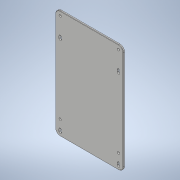
# Autodesk Inventor part: TBD_Box_Fix
Saved by Autodesk Inventor 2021 (Build 250183000, 183)
## iProperties
Created: 2020-10-24
Part Number: TBD_Box_Fix
Material: Generic
Document SubType Name: Modeling
Designer: lgnds
Density: 1 g/cm^3
Appearance: Default
Author: lgnds
Autodesk Inventor part; units mm, degrees
ref_plane "YZ Plane" through (0, 0, 0) normal (1, 0, 0) x (0, 1, 0)
ref_plane "XZ Plane" through (0, 0, 0) normal (0, 1, 0) x (-1, 0, 0)
ref_plane "XY Plane" through (0, 0, 0) normal (0, 0, 1) x (1, 0, 0)
sketch "Sketch1" plane through (0, 0, 0) normal (0, 0, 1) x (1, 0, 0)
  line L0 (-71.5, -114.5) -> (71.5, -114.5)
  line L1 (71.5, -114.5) -> (71.5, 114.5)
  line L2 (71.5, 114.5) -> (-71.5, 114.5)
  line L3 (-71.5, 114.5) -> (-71.5, -114.5)
  line L4 (-71.5, -114.5) -> (71.5, 114.5) construction
  line L5 (71.5, -114.5) -> (-71.5, 114.5) construction
  circle A0 centre (61.5, 105.5) radius 2.5
  line L6 (-147.2223, 0) -> (154.3177, 0) construction
  line L7 (-104.1452, 11) -> (111.2405, 11) construction
  circle A1 centre (61.5, -83.5) radius 2.5
  line L8 (0, 160.3) -> (0, -160.3) construction
  circle A2 centre (-61.5, 105.5) radius 2.5
  circle A3 centre (-61.5, -83.5) radius 2.5
  point P0 (0, 0)
  dimension "d0" = 229
  dimension "d1" = 143
  dimension "d3" = 5
  dimension "d5" = 189
  dimension "d6" = 31
  dimension "d9" = 61.5
  measures "d0" distance of L2.end L0.start
  measures "d1" distance of L1.end L2.end
  measures "d3" diameter of A0
  measures "d5" distance of A1.centre A0.centre
  measures "d6" distance from line of L0 A1.centre
  measures "d9" horizontal distance of point (0, 0) A0.centre
extrude "Plate1" add sketch "Sketch1" along normal blind 3
fillet "Fillet1" radius 10 4 edges at (-71.5, 114.5, 1.5) (71.5, 114.5, 1.5) (71.5, -114.5, 1.5) (-71.5, -114.5, 1.5)
sketch "Sketch2" plane through (0, 0, 3) normal (0, 0, 1) x (1, 0, 0)
  line L0 (-61.5, -107) -> (-61.5, -102) construction
  line L1 (-64, -107) -> (-64, -102)
  line L2 (-59, -102) -> (-59, -107)
  arc A0 (-64, -107) -> (-59, -107) centre (-61.5, -107) ccw
  arc A1 (-59, -102) -> (-64, -102) centre (-61.5, -102) ccw
  line L3 (-93.0799, -19.5) -> (108.9164, -19.5) construction
  line L4 (0, 161.0866) -> (0, -165.0195) construction
  line L5 (-71.5, -104.5) -> (-71.5, 104.5) construction
  line L6 (61.5, -107) -> (61.5, -102) construction
  line L7 (64, -107) -> (64, -102)
  line L8 (59, -102) -> (59, -107)
  arc A2 (59, -107) -> (64, -107) centre (61.5, -107) ccw
  arc A3 (64, -102) -> (59, -102) centre (61.5, -102) ccw
  line L9 (-61.5, 68) -> (-61.5, 63) construction
  line L10 (-64, 68) -> (-64, 63)
  line L11 (-59, 63) -> (-59, 68)
  arc A4 (-59, 68) -> (-64, 68) centre (-61.5, 68) ccw
  arc A5 (-64, 63) -> (-59, 63) centre (-61.5, 63) ccw
  line L12 (61.5, 68) -> (61.5, 63) construction
  line L13 (64, 68) -> (64, 63)
  line L14 (59, 63) -> (59, 68)
  arc A6 (64, 68) -> (59, 68) centre (61.5, 68) ccw
  arc A7 (59, 63) -> (64, 63) centre (61.5, 63) ccw
  line L15 (61.5, -114.5) -> (-61.5, -114.5) projected
  point P0 (0, 0)
  point P1 (-61.5, -104.5)
  point P2 (61.5, -104.5)
  point P3 (71.5, -104.5)
  point P4 (-61.5, 65.5)
  point P5 (-71.5, 65.5)
  point P6 (61.5, 65.5)
  point P7 (71.5, 65.5)
  dimension "d12" = 85
  dimension "d13" = 10
  dimension "d14" = 5
  dimension "d15" = 2.5
  dimension "d18" = 10
  constraints: 34 end point, 24 symmetric about line, 16 point on circle, 8 centre point, 4 tangent, 1 horizontal, 1 midpoint, 1 parallel, 1 vertical, 6 other
  measures "d12" distance from line of L3 point (-61.5, -104.5)
  measures "d13" distance from line of L5 point (-61.5, -104.5)
  measures "d14" distance of L2.start L2.end
  measures "d15" radius of A1
  measures "d18" distance from line of L15 point (-61.5, -104.5)
extrude "Cut1" cut sketch "Sketch2" against normal blind 3
chamfer "Chamfer1" distance 0.75 angle 45 8 edges at (0, -114.5, 3) (-68.5711, -111.5711, 3) (-71.5, 0, 3) (-68.5711, 111.5711, 3) (0, 114.5, 3) (68.5711, 111.5711, 3) (71.5, 0, 3) (68.5711, -111.5711, 3)
equation "\"d18\" = d13"
equation "\"d3\" = d2"
equation "\"d16\" = Thickness"
equation "\"d10\" = Thickness"
equation "\"BendRadius\" = Thickness"
equation "\"BendReliefWidth\" = Thickness"
equation "\"BendReliefDepth\" = 0.5 * Thickness"
equation "\"CornerReliefSize\" = 4 * Thickness"
equation "\"MinimumRemnant\" = 2 * Thickness"
equation "\"TransitionRadius\" = BendRadius"
equation "\"JacobiRadiusSize\" = BendRadius"
equation "\"GapSize\" = Thickness"
equation "\"d2\" = 5"
equation "\"Thickness\" = 3"
body "Solid1"
